Autodesk Inventor part; units mm, degrees
(part 2 of 2)
  line L955 (9.481, 12.2224) -> (9.3887, 12.173)
  line L956 (9.3887, 12.173) -> (9.2008, 12.0779)
  line L957 (9.2008, 12.0779) -> (8.8135, 11.9014)
  line L958 (8.8135, 11.9014) -> (8.4127, 11.7415)
  line L959 (8.4127, 11.7415) -> (7.9999, 11.5967)
  line L960 (7.9999, 11.5967) -> (7.5762, 11.4663)
  line L961 (7.5762, 11.4663) -> (7.1423, 11.3497)
  line L962 (7.1423, 11.3497) -> (6.777, 11.8009)
  line L963 (6.777, 11.8009) -> (6.9813, 12.201)
  line L964 (6.9813, 12.201) -> (7.1969, 12.5884)
  line L965 (7.1969, 12.5884) -> (7.4243, 12.9621)
  line L966 (7.4243, 12.9621) -> (7.6641, 13.3208)
  line L967 (7.6641, 13.3208) -> (7.9172, 13.663)
  line L968 (7.9172, 13.663) -> (8.0493, 13.827)
  line L969 (8.0493, 13.827) -> (8.1169, 13.907)
  line L970 (8.1169, 13.907) -> (8.1855, 13.9856)
  line L971 (8.1855, 13.9856) -> (7.7098, 14.6404)
  line L972 (7.7098, 14.6404) -> (7.6138, 14.5994)
  line L973 (7.6138, 14.5994) -> (7.5168, 14.5599)
  line L974 (7.5168, 14.5599) -> (7.32, 14.4849)
  line L975 (7.32, 14.4849) -> (6.9164, 14.3499)
  line L976 (6.9164, 14.3499) -> (6.5011, 14.2327)
  line L977 (6.5011, 14.2327) -> (6.0755, 14.1319)
  line L978 (6.0755, 14.1319) -> (5.6404, 14.0465)
  line L979 (5.6404, 14.0465) -> (5.1967, 13.9759)
  line L980 (5.1967, 13.9759) -> (4.8805, 14.4628)
  line L981 (4.8805, 14.4628) -> (5.1255, 14.8394)
  line L982 (5.1255, 14.8394) -> (5.3805, 15.2021)
  line L983 (5.3805, 15.2021) -> (5.6457, 15.55)
  line L984 (5.6457, 15.55) -> (5.9217, 15.8817)
  line L985 (5.9217, 15.8817) -> (6.2092, 16.1955)
  line L986 (6.2092, 16.1955) -> (6.3577, 16.3448)
  line L987 (6.3577, 16.3448) -> (6.4333, 16.4173)
  line L988 (6.4333, 16.4173) -> (6.5097, 16.4883)
  line L989 (6.5097, 16.4883) -> (6.1051, 17.1892)
  line L990 (6.1051, 17.1892) -> (6.0053, 17.1585)
  line L991 (6.0053, 17.1585) -> (5.9047, 17.1293)
  line L992 (5.9047, 17.1293) -> (5.7012, 17.0754)
  line L993 (5.7012, 17.0754) -> (5.2857, 16.9833)
  line L994 (5.2857, 16.9833) -> (4.8604, 16.9101)
  line L995 (4.8604, 16.9101) -> (4.4265, 16.8544)
  line L996 (4.4265, 16.8544) -> (3.9849, 16.8149)
  line L997 (3.9849, 16.8149) -> (3.5363, 16.7911)
  line L998 (3.5363, 16.7911) -> (3.2727, 17.3084)
  line L999 (3.2727, 17.3084) -> (3.5558, 17.6573)
  line L1000 (3.5558, 17.6573) -> (3.8472, 17.9913)
  line L1001 (3.8472, 17.9913) -> (4.1474, 18.3096)
  line L1002 (4.1474, 18.3096) -> (4.4565, 18.6106)
  line L1003 (4.4565, 18.6106) -> (4.7752, 18.8927)
  line L1004 (4.7752, 18.8927) -> (4.9385, 19.0256)
  line L1005 (4.9385, 19.0256) -> (5.0212, 19.0899)
  line L1006 (5.0212, 19.0899) -> (5.1047, 19.1525)
  line L1007 (5.1047, 19.1525) -> (4.7756, 19.8919)
  line L1008 (4.7756, 19.8919) -> (4.6731, 19.8717)
  line L1009 (4.6731, 19.8717) -> (4.5701, 19.8532)
  line L1010 (4.5701, 19.8532) -> (4.362, 19.8208)
  line L1011 (4.362, 19.8208) -> (3.9391, 19.7727)
  line L1012 (3.9391, 19.7727) -> (3.5085, 19.7444)
  line L1013 (3.5085, 19.7444) -> (3.0712, 19.7343)
  line L1014 (3.0712, 19.7343) -> (2.6279, 19.7412)
  line L1015 (2.6279, 19.7412) -> (2.1792, 19.7644)
  line L1016 (2.1792, 19.7644) -> (1.9712, 20.3064)
  line L1017 (1.9712, 20.3064) -> (2.2891, 20.6238)
  line L1018 (2.2891, 20.6238) -> (2.6139, 20.9256)
  line L1019 (2.6139, 20.9256) -> (2.9457, 21.2107)
  line L1020 (2.9457, 21.2107) -> (3.2846, 21.4778)
  line L1021 (3.2846, 21.4778) -> (3.631, 21.725)
  line L1022 (3.631, 21.725) -> (3.8074, 21.8401)
  line L1023 (3.8074, 21.8401) -> (3.8963, 21.8954)
  line L1024 (3.8963, 21.8954) -> (3.9859, 21.949)
  line L1025 (3.9859, 21.949) -> (3.7358, 22.7186)
  line L1026 (3.7358, 22.7186) -> (3.6319, 22.7093)
  line L1027 (3.6319, 22.7093) -> (3.5274, 22.7017)
  line L1028 (3.5274, 22.7017) -> (3.3171, 22.6913)
  line L1029 (3.3171, 22.6913) -> (2.8915, 22.6876)
  line L1030 (2.8915, 22.6876) -> (2.4603, 22.7045)
  line L1031 (2.4603, 22.7045) -> (2.0243, 22.7401)
  line L1032 (2.0243, 22.7401) -> (1.5842, 22.7933)
  line L1033 (1.5842, 22.7933) -> (1.1404, 22.8633)
  line L1034 (1.1404, 22.8633) -> (0.9901, 23.4241)
  line L1035 (0.9901, 23.4241) -> (1.3395, 23.7065)
  line L1036 (1.3395, 23.7065) -> (1.6941, 23.9727)
  line L1037 (1.6941, 23.9727) -> (2.0538, 24.2216)
  line L1038 (2.0538, 24.2216) -> (2.4188, 24.4518)
  line L1039 (2.4188, 24.4518) -> (2.7892, 24.6613)
  line L1040 (2.7892, 24.6613) -> (2.9766, 24.7575)
  line L1041 (2.9766, 24.7575) -> (3.0708, 24.8031)
  line L1042 (3.0708, 24.8031) -> (3.1655, 24.847)
  line L1043 (3.1655, 24.847) -> (2.9973, 25.6386)
  line L1044 (2.9973, 25.6386) -> (2.8929, 25.6402)
  line L1045 (2.8929, 25.6402) -> (2.7882, 25.6436)
  line L1046 (2.7882, 25.6436) -> (2.5779, 25.6552)
  line L1047 (2.5779, 25.6552) -> (2.1543, 25.696)
  line L1048 (2.1543, 25.696) -> (1.7273, 25.7578)
  line L1049 (1.7273, 25.7578) -> (1.2974, 25.8389)
  line L1050 (1.2974, 25.8389) -> (0.8652, 25.9378)
  line L1051 (0.8652, 25.9378) -> (0.4312, 26.0538)
  line L1052 (0.4312, 26.0538) -> (0.3404, 26.6272)
  line L1053 (0.3404, 26.6272) -> (0.7173, 26.8716)
  line L1054 (0.7173, 26.8716) -> (1.0978, 27.0992)
  line L1055 (1.0978, 27.0992) -> (1.4816, 27.3091)
  line L1056 (1.4816, 27.3091) -> (1.8686, 27.4999)
  line L1057 (1.8686, 27.4999) -> (2.2589, 27.6697)
  line L1058 (2.2589, 27.6697) -> (2.4553, 27.7456)
  line L1059 (2.4553, 27.7456) -> (2.5538, 27.7812)
  line L1060 (2.5538, 27.7812) -> (2.6526, 27.8149)
  line L1061 (2.6526, 27.8149) -> (2.568, 28.6198)
  line L1062 (2.568, 28.6198) -> (2.4644, 28.6323)
  line L1063 (2.4644, 28.6323) -> (2.3606, 28.6466)
  line L1064 (2.3606, 28.6466) -> (2.1527, 28.6801)
  line L1065 (2.1527, 28.6801) -> (1.7356, 28.765)
  line L1066 (1.7356, 28.765) -> (1.3174, 28.8711)
  line L1067 (1.3174, 28.8711) -> (0.8983, 28.9967)
  line L1068 (0.8983, 28.9967) -> (0.4789, 29.1403)
  line L1069 (0.4789, 29.1403) -> (0.0593, 29.3009)
  line L1070 (0.0593, 29.3009) -> (0.029, 29.8807)
  line L1071 (0.029, 29.8807) -> (0.4294, 30.0843)
  line L1072 (0.4294, 30.0843) -> (0.8316, 30.2709)
  line L1073 (0.8316, 30.2709) -> (1.2352, 30.4396)
  line L1074 (1.2352, 30.4396) -> (1.64, 30.5889)
  line L1075 (1.64, 30.5889) -> (2.0459, 30.7169)
  line L1076 (2.0459, 30.7169) -> (2.2492, 30.772)
  line L1077 (2.2492, 30.772) -> (2.3509, 30.797)
  line L1078 (2.3509, 30.797) -> (2.4527, 30.8203)
  line L1079 (2.4527, 30.8203) -> (2.4527, 31.6296)
  circle A0 centre (31.2249, 31.2249) radius 0.5
  point P0 (0, 0)
  constraints: 2160 end point, 1 centre point
extrude "Extrusion7" add sketch "Sketch7" along normal blind 5
sketch "Sketch8" plane through (0, 5, 0) normal (0, 1, 0) x (1, 0, 0)
  circle A0 centre (-21.2257, -31.351) radius 2.45 projected
  circle A1 centre (-41.2241, -31.0988) radius 2.45 projected
  arc A2 (-31.5371, -33.5546) -> (-30.9715, -33.5617) centre (-31.2508, -33.2754) ccw projected
  line L0 (-30.9715, -33.5617) -> (-28.8952, -31.5371) projected
  arc A3 (-28.8952, -31.5371) -> (-28.8881, -30.9715) centre (-29.1745, -31.2508) ccw projected
  line L1 (-28.8881, -30.9715) -> (-30.9127, -28.8952) projected
  arc A4 (-30.9127, -28.8952) -> (-31.4783, -28.8881) centre (-31.1991, -29.1745) ccw projected
  line L2 (-31.4783, -28.8881) -> (-33.5546, -30.9127) projected
  arc A5 (-33.5546, -30.9127) -> (-33.5617, -31.4783) centre (-33.2754, -31.1991) ccw projected
  line L3 (-33.5617, -31.4783) -> (-31.5371, -33.5546) projected
  circle A6 centre (-31.0988, -21.2257) radius 2.45 projected
  circle A7 centre (-31.351, -41.2241) radius 2.45 projected
  circle A8 centre (-31.2249, -31.2249) radius 15 projected
  point P0 (0, 0)
extrude "Extrusion8" cut sketch "Sketch8" against normal up to next contours A0 | A1 | L3 A5 L2 A4 L1 A3 L0 A2 | A6 | A7
body "Solid2"
